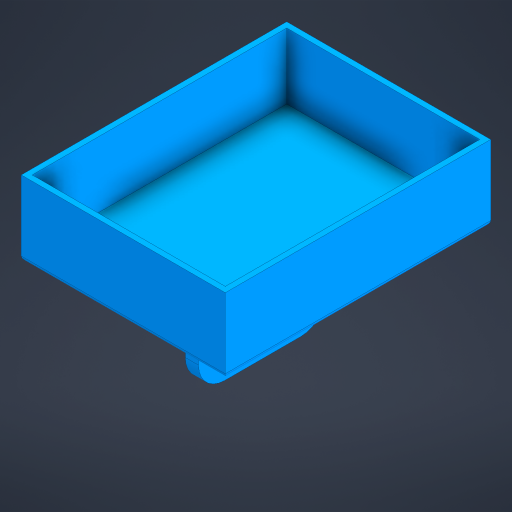
# Autodesk Inventor part: carcasa_pcv
Saved by Autodesk Inventor 2023.1 (Build 271208000, 208)
## iProperties
Created: 2022-11-21
Part Number: carcasa_pcv
Material: Generic
Document SubType Name: Modeling
Designer: amtat
Density: 1 g/cm^3
Appearance: Default
Author: amtat
Autodesk Inventor part; units mm, degrees
ref_plane "YZ Plane" through (0, 0, 0) normal (1, 0, 0) x (0, 1, 0)
ref_plane "XZ Plane" through (0, 0, 0) normal (0, 1, 0) x (-1, 0, 0)
ref_plane "XY Plane" through (0, 0, 0) normal (0, 0, 1) x (1, 0, 0)
sketch "Sketch1" plane through (0, 0, 0) normal (1, 0, 0) x (0, 1, 0)
  circle A0 centre (0, 0) radius 1.6
  line L0 (0, 0) -> (0, -17.3)
  circle A1 centre (0, -17.3) radius 1.6
  line L1 (0, 0) -> (0, 6)
  line L2 (0, -17.3) -> (0, -23.3)
  line L3 (0, 6) -> (-6, 6)
  line L4 (-6, 6) -> (-6, -23.3)
  line L5 (-6, -23.3) -> (0, -23.3)
  line L6 (0, -23.3) -> (16, -23.3)
  line L7 (16, -23.3) -> (16, 6)
  line L8 (16, 6) -> (0, 6)
  dimension "d0" = 3.2
  dimension "d1" = 17.3
  dimension "d2" = 3.2
  dimension "d3" = 6
  dimension "d4" = 6
  dimension "d5" = 6
  dimension "d6" = 16
  constraints: 18 end point, 3 horizontal, 3 perpendicular, 3 vertical, 2 centre point, 2 coincident
  measures "d0" diameter of A0
  measures "d1" distance of L0.start L0.end
  measures "d2" diameter of A1
  measures "d3" distance of L0.start L1.end
  measures "d4" distance of L2.start L2.end
  measures "d5" distance of L1.end L3.end
  measures "d6" distance of L2.end L6.end
extrude "Extrusion1" add sketch "Sketch1" along normal blind 3 contours A0 L1 L8 L7 L6 L2 A1 L0 | A0 L0 A1 L2 L5 L4 L3 L1
sketch "Sketch2" plane through (0, 16, 6) normal (0, 1, 0) x (1, 0, 0)
  line L0 (0, 29.3) -> (0, 0) projected
  line L1 (0, 0) -> (3, 0) projected
  line L2 (3, 29.3) -> (3, 0) projected
  line L3 (0, 29.3) -> (3, 29.3) projected
  line L4 (0, 0) -> (0, 29.3) projected
  line L5 (0, 0) -> (0, 14.6)
  line L6 (0, 14.6) -> (0, -14.4)
  line L7 (0, 14.6) -> (0, 43.6)
  line L8 (0, -14.4) -> (0, -15.65)
  line L9 (0, 43.6) -> (0, 44.85)
  line L10 (0, -15.65) -> (1.5, -15.65)
  line L11 (1.5, -15.65) -> (-20.5, -15.65)
  line L12 (-20.5, -15.65) -> (-20.5, 44.85)
  line L13 (-20.5, 44.85) -> (23.5, 44.85)
  line L14 (23.5, 44.85) -> (23.5, -15.65)
  line L15 (23.5, -15.65) -> (1.5, -15.65)
  line L16 (-20.5, -15.65) -> (-21.75, -15.65)
  line L17 (-21.75, -15.65) -> (-21.75, 46.1)
  line L18 (-21.75, 46.1) -> (23.5, 46.1)
  line L19 (23.5, 46.1) -> (24.75, 46.1)
  line L20 (24.75, 46.1) -> (24.75, -15.65)
  line L21 (24.75, -15.65) -> (23.5, -15.65)
  line L22 (23.5, 44.85) -> (24.75, 44.85)
  line L23 (-20.5, 44.85) -> (-21.75, 44.85)
  point P0 (0, 6)
  dimension "d9" = 14.6
  dimension "d10" = 29
  dimension "d11" = 29
  dimension "d12" = 1.25
  dimension "d13" = 1.25
  dimension "d14" = 22
  dimension "d15" = 44
  dimension "d16" = 90
  dimension "d17" = 1.25
  dimension "d18" = 61.75
  dimension "d19" = 1.25
  constraints: 38 end point, 9 point on line, 7 perpendicular, 3 vertical, 2 horizontal, 1 parallel
  measures "d9" distance of L0.end L5.end
  measures "d10" distance of L5.end L6.end
  measures "d11" distance of L5.end L7.end
  measures "d12" distance of L6.end L8.end
  measures "d13" distance of L7.end L9.end
  measures "d14" distance of L10.end L11.end
  measures "d15" distance of L12.end L13.end
  measures "d16" angle of L12 L13
  measures "d17" distance of L11.end L16.end
  measures "d18" distance of L16.end L17.end
  measures "d19" distance of L18.end L19.end
extrude "Extrusion2" add sketch "Sketch2" along normal blind 2 contours L3 L2 L1 L0 | L7 L9 L13 L14 L15 L10 L8 L6 L1 L2 L3 | L0 L6 L8 L11 L12 L13 L9 L7 | L12 L16 L17 L23 | L22 L20 L21 L14
sketch "Sketch3" plane through (0, 18, 6) normal (0, 1, 0) x (1, 0, 0)
  line L0 (24.75, 44.85) -> (-21.75, 44.85) projected
  line L1 (-21.75, 44.85) -> (-21.75, -15.65) projected
  line L2 (-21.75, -15.65) -> (24.75, -15.65) projected
  line L3 (24.75, -15.65) -> (24.75, 44.85) projected
  line L4 (-21.75, -15.65) -> (24.75, -15.65) projected
  line L5 (24.75, -15.65) -> (24.75, -14.4)
  line L6 (24.75, -15.65) -> (24.75, 44.85) projected
  line L7 (24.75, -14.4) -> (-20.5, -14.4)
  line L8 (-20.5, -14.4) -> (-20.5, 43.6)
  line L9 (-20.5, 43.6) -> (23.5, 43.6)
  line L10 (23.5, 43.6) -> (23.5, -14.4)
  point P0 (0, 6)
  dimension "d22" = 1.25
  dimension "d23" = 45.25
  dimension "d24" = 58
  dimension "d25" = 44
  constraints: 10 end point, 4 perpendicular, 2 point on line
  measures "d22" distance of L2.end L5.end
  measures "d23" distance of L5.end L7.end
  measures "d24" distance of L7.end L8.end
  measures "d25" distance of L8.end L9.end
extrude "Extrusion3" add sketch "Sketch3" along normal blind 15
fillet "Fillet1" radius 1 4 edges at (3, 16, -8.65) (1.5, 16, -23.3) (0, 16, -8.65) (1.5, 16, 6)
fillet "Fillet2" radius 6 2 edges at (1.5, -6, 6) (1.5, -6, -23.3)
fillet "Fillet3" radius 1 4 edges at (1.5, 16, -38.85) (24.75, 16, -8.6) (-21.75, 16, -8.6) (1.5, 16, 21.65)
body "Solid1"
